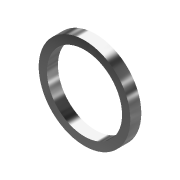
# Autodesk Inventor part: 00_Ringmagnet_25mm
Saved by Autodesk Inventor 2019.4 (Build 234330000, 330)
## iProperties
Created: 2020-10-23
Part Number: 00_Ringmagnet_25mm
Material: Generic
Document SubType Name: Modeling
Designer: diederichbenedict
Density: 1 g/cm^3
Appearance: Chrome - Polished
Author: diederichbenedict
Autodesk Inventor part; units mm, degrees
ref_plane "YZ Plane" through (0, 0, 0) normal (1, 0, 0) x (0, 1, 0)
ref_plane "XZ Plane" through (0, 0, 0) normal (0, 1, 0) x (-1, 0, 0)
ref_plane "XY Plane" through (0, 0, 0) normal (0, 0, 1) x (1, 0, 0)
sketch "Sketch1" plane through (0, 0, 0) normal (0, 0, 1) x (1, 0, 0)
  circle A0 centre (0, 0) radius 12.5
  circle A1 centre (0, 0) radius 10.25
  dimension "d0" = 25
  dimension "d1" = 20.5
  constraints: 2 centre point, 2 coincident
  measures "d0" diameter of A0
  measures "d1" diameter of A1
extrude "Extrusion1" add sketch "Sketch1" along normal blind 3
sketch "Sketch2" plane through (0, 0, 0) normal (0, 0, -1) x (-1, 0, 0)
  circle A0 centre (0, 0) radius 6 construction
  circle A1 centre (0, 0) radius 10.25 construction
  circle A2 centre (0, 0) radius 6.1
  circle A3 centre (0, 0) radius 10.2
  circle A4 centre (0, 0) radius 7
  circle A5 centre (0, 0) radius 9.25
  point P0 (0, 0)
  dimension "d4" = 12.2
  dimension "d5" = 20.4
  dimension "d6" = 14
  dimension "d7" = 18.5
  constraints: 4 centre point, 4 coincident
  measures "d4" diameter of A2
  measures "d5" diameter of A3
  measures "d6" diameter of A4
  measures "d7" diameter of A5
body "Solid1"
